Test roulement (Autodesk Fusion 360 design; units mm, degrees)
Autodesk Fusion 360 part; units mm, degrees
sketch "Sketch1" plane through (0, 0, 0) normal (0, 0, 1) x (1, 0, 0)
  circle A0 centre (0, 0) radius 11.05
  circle A1 centre (0, 0) radius 13.75
  circle A2 centre (0, 0) radius 9.05
  dimension "d1" = 22.1
  dimension "d2" = 27.5
  dimension "d3" = -2
  constraint coincident A0.centre A1.centre
  measures "d1" diameter of A0
  measures "d2" diameter of A1
extrude "Extrude1" add sketch "Sketch1" along normal blind 10 contours A0 makes body 1
extrude "Extrude2" add sketch "Sketch1" along normal blind 17 contours A1 bodies 1
sketch "Sketch2" plane through (0, 0, 0) normal (0, 0, 1) x (1, 0, 0)
  circle A0 centre (0, 0) radius 4
  circle A1 centre (0, 0) radius 7.5
  circle A2 centre (0, 0) radius 2.65
  circle A3 centre (0, 0) radius 5
  line L0 (-1.1236, 2.4) -> (1.1236, 2.4)
  line L1 (10, -2.5) -> (-28.5, -2.5)
  line L2 (-30, -1) -> (-30, 1)
  line L3 (-28.5, 2.5) -> (10, 2.5)
  line L4 (30, 0) -> (10, 2.5)
  line L5 (30, 0) -> (10, -2.5)
  line L6 (10, 2.5) -> (10, 3.4574) construction
  line L7 (10, -3.4574) -> (10, -2.5) construction
  line L8 (0, 0) -> (-30, 0) construction
  line L9 (0, 0) -> (30, 0) construction
  arc A4 (-28.5, 2.5) -> (-30, 1) centre (-28.5, 1) ccw
  arc A5 (-30, -1) -> (-28.5, -2.5) centre (-28.5, -1) ccw
  line L10 (-15, 1.5) -> (-25, 1.5)
  arc A6 (-25, 1.5) -> (-25, -1.5) centre (-25, 0) ccw
  line L11 (-25, -1.5) -> (-15, -1.5)
  arc A7 (-15, -1.5) -> (-15, 1.5) centre (-15, 0) ccw
  line L12 (-15, 0) -> (-25, 0) construction
  point P0 (-30, -2.5)
  point P1 (-30, 2.5)
  point P2 (-20, 0)
  dimension "d8" = 8
  dimension "d9" = 15
  dimension "d10" = 5.3
  dimension "d11" = 1
  dimension "d18" = 2.4
  dimension "d25" = 30
  dimension "d26" = 30
  dimension "d27" = 20
  dimension "d30" = 1.5
  dimension "d31" = 1.5
  dimension "d32" = 1.5
  dimension "d33" = 10
  dimension "d34" = 10
  dimension "d35" = 2.5
  dimension "d36" = 2.5
  constraint coincident A0.centre A1.centre
  constraint concentric A1 A2
  constraint coincident A2 L0.start
  constraint coincident A2 L0.end
  constraint horizontal L0
  constraint perpendicular L1 L2
  constraint parallel L1 L3
  constraint horizontal L1
  constraint perpendicular L1 L6
  constraint collinear L6 L7
  constraint perpendicular L2 L8
  constraint horizontal L9
  constraint coincident L2 L8.end
  constraint coincident P1 L3
  constraint coincident P1 L2
  constraint tangent L3 A4
  constraint tangent L2 A4
  constraint coincident P0 L2
  constraint coincident P0 L1
  constraint tangent L2 A5
  constraint tangent L1 A5
  constraint tangent L10 A6
  constraint tangent A6 L11
  constraint parallel L10 L11
  constraint tangent L11 A7
  constraint tangent L10 A7
  constraint parallel L8 L12
  constraint midpoint L12 P2
  constraint coincident L8 P2
  measures "d8" diameter of A0
  measures "d9" diameter of A1
  measures "d10" diameter of A2
  measures "d18" distance of A0.centre L0
  measures "d25" distance of A0.centre L4.start
  measures "d26" distance of A0.centre L8.end
  measures "d27" horizontal distance of L4.start L3.end
  measures "d30" radius of A4
  measures "d31" radius of A5
  measures "d32" radius of A6
  measures "d33" distance of A7.centre A6.centre
  measures "d34" distance of L8.end P2
  measures "d35" distance of L3 A0.centre
  measures "d36" distance of L1 A0.centre
extrude "Extrude3" add sketch "Sketch2" along normal blind 5 separate body contours A0 A2 L1 L3 | A0 A2 L3 | A0 A2 L1 | A0 A2 L1 L3 | A2 L3 | A2 L0 L3 makes body 2
extrude "Extrude4" add sketch "Sketch2" along normal blind 3 contours A0 A3 L1 L3 | A0 A3 L3 | A0 A3 L1 | A0 A3 L1 L3 bodies 2
extrude "Extrude5" add sketch "Sketch2" along normal blind 2 contours A0 A2 L1 L3 | A0 A3 L1 L3 | A0 A2 L3 | A0 A3 L3 | A0 A3 L1 | A0 A2 L1 | A0 A2 L1 L3 | A0 A3 L1 L3 | A2 L3 | A2 L0 L3 | A1 A3 L1 L3 | A1 A3 L3 | A1 A3 L1 | A2 L1 | A1 A3 L1 L3 | A1 L1 L3 L4 L5 | A1 L1 L2 L3 A4 A5 bodies 2
move_body "Move2" bodies 1 to x (1, 0, 0) y (0, 1, 0) z (0, 0, 1) at (0, 42, 0)
move_body "Move1" [suppressed]
hidden bodies 1
